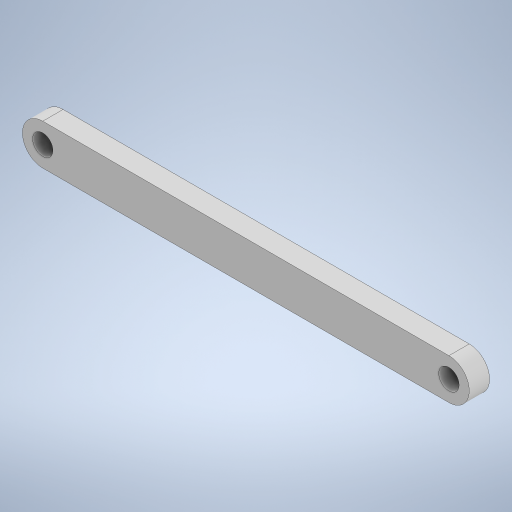
# Autodesk Inventor part: AB
Saved by Autodesk Inventor 2024 (Build 280153000, 153)
## iProperties
Created: 2025-09-18
Part Number: AB
Material: Generic
Document SubType Name: Modeling
Designer: Hello
Density: 1 g/cm^3
Appearance: Default
Author: Hello
Autodesk Inventor part; units mm, degrees
ref_plane "YZ Plane" through (0, 0, 0) normal (1, 0, 0) x (0, 1, 0)
ref_plane "XZ Plane" through (0, 0, 0) normal (0, 1, 0) x (-1, 0, 0)
ref_plane "XY Plane" through (0, 0, 0) normal (0, 0, 1) x (1, 0, 0)
sketch "Sketch1" plane through (0, 0, 0) normal (0, 0, 1) x (1, 0, 0)
  circle A0 centre (0, 0) radius 5
  arc A1 (0, 10) -> (0, -10) centre (0, 0) ccw
  line L0 (0, 0) -> (200, 0)
  circle A2 centre (200, 0) radius 5
  arc A3 (200, -10) -> (200, 10) centre (200, 0) ccw
  line L1 (0, 10) -> (200, 10)
  line L2 (0, -10) -> (200, -10)
  dimension "d0" = 10
  dimension "d1" = 20
  dimension "d2" = 200
  dimension "d3" = 10
  dimension "d4" = 20
  constraints: 6 end point, 4 centre point, 4 point on circle, 3 coincident, 2 tangent, 1 horizontal
  measures "d0" diameter of A0
  measures "d1" diameter of A1
  measures "d2" distance of L0.start L0.end
  measures "d3" diameter of A2
  measures "d4" diameter of A3
extrude "Extrusion1" add sketch "Sketch1" along normal blind 10
body "Solid1"
